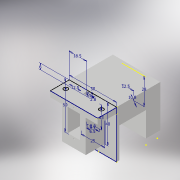
# Autodesk Inventor part: servo_holder
Saved by Autodesk Inventor 2021 (Build 250183000, 183)
## iProperties
Created: 2020-03-14
Part Number: servo_holder
Material: Generic
Document SubType Name: Modeling
Designer: Mazur
Density: 1 g/cm^3
Appearance: Default
Author: Mazur
Autodesk Inventor part; units mm, degrees
note: some values were not read from the file. Chosen so that the rebuilt part matches the saved one: direction of "Hole1".
ref_plane "YZ Plane" through (0, 0, 0) normal (1, 0, 0) x (0, 1, 0)
ref_plane "XZ Plane" through (0, 0, 0) normal (0, 1, 0) x (-1, 0, 0)
ref_plane "XY Plane" through (0, 0, 0) normal (0, 0, 1) x (1, 0, 0)
sketch "Sketch1" plane through (0, 0, 0) normal (0, 0, 1) x (1, 0, 0)
  point P0 (0, 0)
sketch "Sketch2" plane through (0, 0, 0) normal (0, 0, 1) x (1, 0, 0)
  line L0 (0, 0) -> (-50, 0)
  line L1 (0, 0) -> (-50, 0)
  line L2 (0, 0) -> (-50, 0)
  line L3 (-50, 0) -> (-50, 50)
  line L4 (-50, 50) -> (0, 50)
  line L5 (0, 50) -> (0, 0)
  line L6 (-31.5, 44) -> (-18.5, 44)
  line L7 (-18.5, 44) -> (-18.5, 21)
  line L8 (-18.5, 21) -> (-31.5, 21)
  line L9 (-31.5, 21) -> (-31.5, 44)
  circle A0 centre (-25, 46.8) radius 0.75
  circle A1 centre (-25, 18.2) radius 0.75
  line L10 (-37.5, 50) -> (-12.5, 50)
  line L11 (-12.5, 50) -> (-12.5, 10)
  line L12 (-12.5, 10) -> (-37.5, 10)
  line L13 (-37.5, 10) -> (-37.5, 50)
  line L14 (-37.5, 44) -> (-50, 44)
  line L15 (-12.5, 44) -> (0, 44)
  dimension "d4" = 50
  dimension "d5" = 50
  dimension "d6" = 13
  dimension "d7" = 23
  dimension "d8" = 18.5
  dimension "d9" = 6
  dimension "d10" = 1.5
  dimension "d11" = 6.5
  dimension "d12" = 2.8
  dimension "d13" = 1.5
  dimension "d14" = 6.5
  dimension "d15" = 2.8
  dimension "d16" = 25
  dimension "d17" = 40
  dimension "d18" = 12.5
  constraints: 32 end point, 7 point on line, 6 parallel, 5 horizontal, 4 perpendicular, 2 centre point
  measures "d4" distance of L3.end L4.end
  measures "d5" distance of L2.end L3.end
  measures "d6" distance of L7.end L8.end
  measures "d7" distance of L6.end L7.end
  measures "d8" horizontal distance of L6.start L3.end
  measures "d9" vertical distance of L3.end L6.start
  measures "d10" diameter of A0
  measures "d11" horizontal distance of A0.centre L6.start
  measures "d12" vertical distance of A0.centre L6.start
  measures "d13" diameter of A1
  measures "d14" horizontal distance of L8.end A1.centre
  measures "d15" vertical distance of L7.end A1.centre
  measures "d16" distance of L11.end L12.end
  measures "d17" distance of L10.end L11.end
  measures "d18" distance between parallel lines of L3 L13
extrude "Extrusion1" add sketch "Sketch2" along normal blind 20 contours L11 L12 L13 L4
extrude "Extrusion2" add sketch "Sketch2" along normal blind 3 contours L6 L7 L8 L9
extrude "Extrusion3" add sketch "Sketch2" against normal blind 3 contours L0 L3 L14 L13 L12 L11 L15 L5 | L15 L11 L4 L5 | L3 L4 L13 L14
extrude "Extrusion4" add sketch "Sketch2" against normal blind 3 contours L11 L12 L13 L4
extrude "Extrusion5" add sketch "Sketch2" against normal blind 3 contours L6 L7 L8 L9
sketch "Sketch3" plane through (-18.5, 21, 20) normal (-1, 0, 0) x (0, 0, 1)
  point P0 (-20, -21)
sketch "Sketch4" plane through (0, 0, -3) normal (0, 0, -1) x (-1, 0, 0)
  line L0 (12.5, 50) -> (37.5, 50) projected
  line L1 (37.5, 50) -> (37.5, 10) projected
  line L2 (12.5, 50) -> (37.5, 50)
  line L3 (37.5, 50) -> (37.5, 35.8782)
  line L4 (37.5, 35.8782) -> (12.5, 35.8782)
  line L5 (12.5, 35.8782) -> (12.5, 50)
  point P0 (0, 0)
  constraints: 8 end point, 2 parallel, 1 horizontal, 1 perpendicular, 1 point on line
extrude "Extrusion6" add sketch "Sketch4" along normal blind 40
sketch "Sketch5" plane through (-37.5, 35.8782, -3) normal (0, -1, 0) x (1, 0, 0)
  line L0 (0, -40) -> (25, -40) projected
  line L1 (25, -40) -> (0, -40)
  line L2 (0, -40) -> (0, -28)
  line L3 (0, -28) -> (25, -28)
  line L4 (25, -28) -> (25, -40)
  point P0 (37.5, 3)
  dimension "d31" = 25
  dimension "d32" = 12
  constraints: 8 end point, 2 parallel, 1 horizontal, 1 perpendicular
  measures "d31" distance of L2.end L3.end
  measures "d32" distance of L1.end L2.end
extrude "Extrusion7" add sketch "Sketch5" along normal blind 30
sketch "Sketch6" plane through (0, 0, -43) normal (0, 0, -1) x (-1, 0, 0)
  circle A0 centre (25, 22) radius 5.4
  line L0 (37.5, 50) -> (12.5, 50) projected
  line L1 (37.5, 50) -> (37.5, 5.8782) projected
  point P0 (0, 0)
  dimension "d35" = 10.8
  dimension "d36" = 28
  dimension "d37" = 12.5
  constraints: 1 centre point
  measures "d35" diameter of A0
  measures "d36" distance from line of A0.centre L0
  measures "d37" distance from line of L1 A0.centre
hole "Hole1" at (-25, 22, -43) direction (0, 0, 1) diameter 10.8 depth 12
sketch "Sketch7" plane through (-37.5, 50, 20) normal (0, 1, 0) x (1, 0, 0)
  line L0 (0, 20) -> (25, 20) projected
  line L1 (7.5, 20) -> (17.5, 20)
  line L2 (17.5, 20) -> (17.5, 15)
  line L3 (17.5, 15) -> (7.5, 15)
  line L4 (7.5, 15) -> (7.5, 20)
  line L5 (0, 20) -> (0, 0) projected
  point P0 (37.5, 20)
  dimension "d47" = 10
  dimension "d48" = 5
  dimension "d49" = 7.5
  constraints: 8 end point, 2 parallel, 1 horizontal, 1 perpendicular, 1 point on line
  measures "d47" distance of L2.end L3.end
  measures "d48" distance of L1.end L2.end
  measures "d49" distance between parallel lines of L5 L4
extrude "Extrusion8" cut sketch "Sketch7" against normal blind 10
extrude "Extrusion9" cut sketch "Sketch2" against normal blind 2 contours L6 L7 L8 L9
extrude "Extrusion10" cut sketch "Sketch2" along normal blind 3 contours L6 L7 L8 L9
extrude "Extrusion11" add sketch "Sketch2" against normal blind 3 contours L6 L7 L8 L9
extrude "Extrusion12" cut sketch "Sketch2" against normal blind 4 contours L6 L7 L8 L9
thicken "Thicken1" operation add thickness 12.5 both sides no extend neighbours yes toward (1, 0, 0) faces at (-12.5, 45.2927, -25.6667)
thicken "Thicken2" operation add thickness 12.5 both sides no extend neighbours yes toward (-1, 0, 0) faces at (-37.5, 45.2927, -25.6667)
thicken "Thicken3" operation add thickness 0.5 both sides no extend neighbours yes toward (0, -1, 0) faces at (-27.1667, 21, 12.3333)
thicken "Thicken4" operation add thickness 0.5 both sides no extend neighbours yes toward (0, 1, 0) faces at (-26.6667, 44, 15)
sketch "Sketch8" plane through (0, 5.8782, -31) normal (0, 0, 1) x (1, 0, 0)
  point P0 (0, -5.8782)
sketch "Sketch9" plane through (0, 5.8782, -31) normal (0, 0, 1) x (1, 0, 0)
  circle A0 centre (-25, 16.1218) radius 5.4 projected
  circle A1 centre (-25, 16.1218) radius 9.9
  line L0 (-25, 6.2218) -> (-33.5737, 11.1718)
  line L1 (-33.5737, 11.1718) -> (-33.5737, 21.0718)
  line L2 (-33.5737, 21.0718) -> (-25, 26.0218)
  line L3 (-25, 26.0218) -> (-16.4263, 21.0718)
  line L4 (-16.4263, 21.0718) -> (-16.4263, 11.1718)
  line L5 (-16.4263, 11.1718) -> (-25, 6.2218)
  point P0 (0, -5.8782)
  dimension "d68" = 19.8
  constraints: 12 end point, 2 coincident, 1 vertical alignment, 15 other
extrude "Extrusion13" cut sketch "Sketch9" against normal blind 6.8 contours A0 | L4 L5 L0 L1 L2 L3
thicken "Thicken5" operation add thickness 3.978 both sides no extend neighbours yes toward (0, -1, 0) faces at (-22.8333, 35.8782, -22)
thicken "Thicken6" operation add thickness 3 both sides no extend neighbours yes toward (0, 0, -1) faces at (-25, 42.4667, -43)
extrude "Extrusion14" add sketch "Sketch2" along normal up to surface (20 mm away) contours L15 L11 L4 L5 | L3 L4 L13 L14
sketch "Sketch10" plane through (-50, 44, 20) normal (0, -1, 0) x (1, 0, 0)
  point P0 (50, -20)
sketch "Sketch11" plane through (-50, 44, 20) normal (0, -1, 0) x (1, 0, 0)
  line L0 (12.5, -20) -> (0, 0)
  line L1 (12.5, 0) -> (12.5, -20) projected
  line L2 (12.5, 0) -> (0, -20)
  point P0 (50, -20)
  point P1 (6.25, -10)
  constraints: 4 end point, 1 midpoint
hole "Hole2" at (-43.75, 44, 10) direction (0, 1, 0) diameter 4.3 end through all
sketch "Sketch12" plane through (-12.5, 44, 20) normal (0, -1, 0) x (1, 0, 0)
  line L0 (0, -20) -> (0, 0) projected
  line L1 (12.5, -20) -> (0, 0)
  line L2 (12.5, 0) -> (0, -20)
  point P0 (6.25, -10)
  constraints: 4 end point, 1 midpoint
hole "Hole3" at (-6.25, 44, 10) direction (0, 1, 0) diameter 4.3 end through all
sketch "Sketch13" plane through (-50, 50, 20) normal (0, 1, 0) x (1, 0, 0)
  circle A0 centre (6.25, 10) radius 2.15 projected
  circle A1 centre (6.25, 10) radius 2.15
  circle A2 centre (43.75, 10) radius 2.15 projected
  circle A3 centre (43.75, 10) radius 2.15
  line L0 (-0.0918, 20) -> (50, 20)
  line L1 (50, 20) -> (50, 0)
  line L2 (50, 0) -> (-0.0918, 0)
  line L3 (-0.0918, 0) -> (-0.0918, 20)
  constraints: 8 end point, 2 centre point, 2 coincident, 2 parallel, 1 horizontal, 1 perpendicular
body "Solid1"
